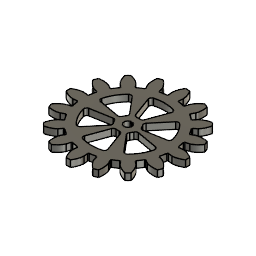
Gear 1 (Autodesk Fusion 360 design; units mm, degrees)
description: Spur Gear; Module: 12.700000; Num Teeth: 16; Pressure Angle: 20.000000; Backlash: 0.00 mm
Autodesk Fusion 360 part; units mm, degrees
sketch "Sketch1" plane through (0, 0, 0) normal (0, 0, 1) x (1, 0, 0) in component "Spur Gear (16 teeth)"
  circle A0 centre (0, 0) radius 86.3092
  circle A1 centre (0, 0) radius 6.35
extrude "Extrude1" add sketch "Sketch1" along normal blind 12.7 in component "Spur Gear (16 teeth)"
sketch "Sketch2" plane through (0, 0, 0) normal (0, 0, 1) x (1, 0, 0) in component "Spur Gear (16 teeth)"
  spline S0 degree 5 poles (94.863, -10.773) (94.919, -10.7793) (95.0311, -10.7904) (95.1995, -10.8021) (95.4243, -10.8085) (95.706, -10.8038) (95.9881, -10.7901) (96.2705, -10.7709) (96.5529, -10.7488) (96.8354, -10.7247) (97.1179, -10.6983) (97.4005, -10.669) (97.683, -10.6358) (97.9655, -10.5982) (98.2481, -10.5561) (98.5306, -10.51) (98.813, -10.4605) (99.0953, -10.4081) (99.3775, -10.3532) (99.6596, -10.2959) (99.9416, -10.2361) (100.2234, -10.1738) (100.505, -10.1088) (100.7865, -10.041) (101.0678, -9.9705) (101.3489, -9.8975) (101.6299, -9.8219) (101.9106, -9.7441) (102.1911, -9.664) (102.4714, -9.5816) (102.7515, -9.4971) (103.0313, -9.4104) (103.3109, -9.3215) (103.5902, -9.2304) (103.8693, -9.1372) (104.1481, -9.0418) (104.4266, -8.9443) (104.7048, -8.8449) (104.9828, -8.7434) (105.2604, -8.6399) (105.5378, -8.5345) (105.8149, -8.4272) (106.0916, -8.3179) (106.368, -8.2067) (106.6441, -8.0937) (106.9199, -7.9787) (107.1953, -7.8619) (107.4704, -7.7433) (107.7452, -7.6229) (108.0196, -7.5007) (108.2936, -7.3767) (108.5673, -7.2509) (108.8406, -7.1234) (109.1135, -6.9942) (109.3861, -6.8632) (109.6583, -6.7306) (109.93, -6.5962) (110.2014, -6.4602) (110.4724, -6.3225) (110.743, -6.1831) (111.0132, -6.0422) (111.283, -5.8995) (111.5523, -5.7553) (111.8213, -5.6095) (112.0898, -5.4621) (112.3578, -5.3131) (112.6255, -5.1625) (112.8927, -5.0104) (113.1594, -4.8567) (113.4257, -4.7015) (113.6916, -4.5447) (113.9039, -4.4181) (114.063, -4.3224) (114.1689, -4.2584) (114.2218, -4.2262) knots 0 0 0 0 0 0 0.01428571 0.02857143 0.04285714 0.05714286 0.07142857 0.08571429 0.1 0.11428571 0.12857143 0.14285714 0.15714286 0.17142857 0.18571429 0.2 0.21428571 0.22857143 0.24285714 0.25714286 0.27142857 0.28571429 0.3 0.31428571 0.32857143 0.34285714 0.35714286 0.37142857 0.38571429 0.4 0.41428571 0.42857143 0.44285714 0.45714286 0.47142857 0.48571429 0.5 0.51428571 0.52857143 0.54285714 0.55714286 0.57142857 0.58571429 0.6 0.61428571 0.62857143 0.64285714 0.65714286 0.67142857 0.68571429 0.7 0.71428571 0.72857143 0.74285714 0.75714286 0.77142857 0.78571429 0.8 0.81428571 0.82857143 0.84285714 0.85714286 0.87142857 0.88571429 0.9 0.91428571 0.92857143 0.94285714 0.95714286 0.97142857 0.98571429 1 1 1 1 1 1
  spline S1 degree 5 poles (94.863, 10.773) (94.919, 10.7793) (95.0311, 10.7904) (95.1995, 10.8021) (95.4243, 10.8085) (95.706, 10.8038) (95.9881, 10.7901) (96.2705, 10.7709) (96.5529, 10.7488) (96.8354, 10.7247) (97.1179, 10.6983) (97.4005, 10.669) (97.683, 10.6358) (97.9655, 10.5982) (98.2481, 10.5561) (98.5306, 10.51) (98.813, 10.4605) (99.0953, 10.4081) (99.3775, 10.3532) (99.6596, 10.2959) (99.9416, 10.2361) (100.2234, 10.1738) (100.505, 10.1088) (100.7865, 10.041) (101.0678, 9.9705) (101.3489, 9.8975) (101.6299, 9.8219) (101.9106, 9.7441) (102.1911, 9.664) (102.4714, 9.5816) (102.7515, 9.4971) (103.0313, 9.4104) (103.3109, 9.3215) (103.5902, 9.2304) (103.8693, 9.1372) (104.1481, 9.0418) (104.4266, 8.9443) (104.7048, 8.8449) (104.9828, 8.7434) (105.2604, 8.6399) (105.5378, 8.5345) (105.8149, 8.4272) (106.0916, 8.3179) (106.368, 8.2067) (106.6441, 8.0937) (106.9199, 7.9787) (107.1953, 7.8619) (107.4704, 7.7433) (107.7452, 7.6229) (108.0196, 7.5007) (108.2936, 7.3767) (108.5673, 7.2509) (108.8406, 7.1234) (109.1135, 6.9942) (109.3861, 6.8632) (109.6583, 6.7306) (109.93, 6.5962) (110.2014, 6.4602) (110.4724, 6.3225) (110.743, 6.1831) (111.0132, 6.0422) (111.283, 5.8995) (111.5523, 5.7553) (111.8213, 5.6095) (112.0898, 5.4621) (112.3578, 5.3131) (112.6255, 5.1625) (112.8927, 5.0104) (113.1594, 4.8567) (113.4257, 4.7015) (113.6916, 4.5447) (113.9039, 4.4181) (114.063, 4.3224) (114.1689, 4.2584) (114.2218, 4.2262) knots 0 0 0 0 0 0 0.01428571 0.02857143 0.04285714 0.05714286 0.07142857 0.08571429 0.1 0.11428571 0.12857143 0.14285714 0.15714286 0.17142857 0.18571429 0.2 0.21428571 0.22857143 0.24285714 0.25714286 0.27142857 0.28571429 0.3 0.31428571 0.32857143 0.34285714 0.35714286 0.37142857 0.38571429 0.4 0.41428571 0.42857143 0.44285714 0.45714286 0.47142857 0.48571429 0.5 0.51428571 0.52857143 0.54285714 0.55714286 0.57142857 0.58571429 0.6 0.61428571 0.62857143 0.64285714 0.65714286 0.67142857 0.68571429 0.7 0.71428571 0.72857143 0.74285714 0.75714286 0.77142857 0.78571429 0.8 0.81428571 0.82857143 0.84285714 0.85714286 0.87142857 0.88571429 0.9 0.91428571 0.92857143 0.94285714 0.95714286 0.97142857 0.98571429 1 1 1 1 1 1
  arc A0 (114.2218, -4.2262) -> (114.2218, 4.2262) centre (0, 0) ccw
  line L0 (85.748, -9.739) -> (94.863, -10.773)
  line L1 (85.748, 9.739) -> (94.863, 10.773)
  line L2 (85.748, -9.739) -> (85.748, 9.739)
  point P0 (96.2162, -10.774)
  point P1 (97.5833, -10.647)
  point P2 (98.9587, -10.4331)
  point P3 (100.3403, -10.1465)
  point P4 (101.7263, -9.7949)
  point P5 (103.1155, -9.3833)
  point P6 (104.5068, -8.9153)
  point P7 (105.8991, -8.3936)
  point P8 (107.2914, -7.8202)
  point P9 (108.6828, -7.1968)
  point P10 (110.0724, -6.5246)
  point P11 (111.4593, -5.8049)
  point P12 (112.8428, -5.0385)
  point P13 (96.2162, 10.774)
  point P14 (97.5833, 10.647)
  point P15 (98.9587, 10.4331)
  point P16 (100.3403, 10.1465)
  point P17 (101.7263, 9.7949)
  point P18 (103.1155, 9.3833)
  point P19 (104.5068, 8.9153)
  point P20 (105.8991, 8.3936)
  point P21 (107.2914, 7.8202)
  point P22 (108.6828, 7.1968)
  point P23 (110.0724, 6.5246)
  point P24 (111.4593, 5.8049)
  point P25 (112.8428, 5.0385)
extrude "Extrude2" add sketch "Sketch2" along normal blind 12.7 in component "Spur Gear (16 teeth)"
fillet "Fillet1" radius 1.5875 2 edges at (85.7578, -9.7401, 6.35) (85.7578, 9.7401, 6.35) in component "Spur Gear (16 teeth)"
pattern_circular "C-Pattern1" count 16 over 360 about axis through (0, 0, 0) along (0, 0, 1) of "Extrude2", "Fillet1" in component "Spur Gear (16 teeth)"
sketch "Sketch3" plane through (0, 0, 0) normal (0, 0, 1) x (1, 0, 0) in component "Spur Gear (16 teeth)"
  circle A0 centre (0, 0) radius 101.6 construction
sketch "Sketch1 (2)" plane through (0, 0, 0) normal (0, 0, 1) x (1, 0, 0)
  circle A0 centre (0, 0) radius 7.55
  line L0 (0, 13) -> (0, -11)
  line L1 (1.4, 7.4191) -> (1.4, 5.65)
  line L2 (1.4, 5.65) -> (-1.4, 5.65)
  line L3 (-1.4, 5.65) -> (-1.4, 7.4191)
  circle A1 centre (0, 0) radius 70
  circle A2 centre (0, 0) radius 20
  line L4 (0, 0) -> (-6.8404, 18.7939)
  line L5 (0, 0) -> (6.8404, 18.7939)
  line L6 (-6.8404, 18.7939) -> (-23.9414, 65.7785)
  line L7 (6.8404, 18.7939) -> (23.9414, 65.7785)
  line L8 (-19.6962, 3.473) -> (-68.9365, 12.1554)
  line L9 (-12.8558, 15.3209) -> (-44.9951, 53.6231)
  line L10 (-12.8558, -15.3209) -> (-44.9951, -53.6231)
  line L11 (-19.6962, -3.473) -> (-68.9365, -12.1554)
  line L12 (6.8404, -18.7939) -> (23.9414, -65.7785)
  line L13 (-6.8404, -18.7939) -> (-23.9414, -65.7785)
  line L14 (19.6962, -3.473) -> (68.9365, -12.1554)
  line L15 (12.8558, -15.3209) -> (44.9951, -53.6231)
  line L16 (12.8558, 15.3209) -> (44.9951, 53.6231)
  line L17 (19.6962, 3.473) -> (68.9365, 12.1554)
  point P0 (0, 7.55)
  dimension "d17" = 15.1
  dimension "d18" = 2.8
  dimension "d19" = 1.9
  dimension "d24" = -50
  dimension "d25" = 40
  dimension "d26" = 40
  dimension "d28" = 20
  dimension "d30" = 360
  constraint coincident A0.centre A1.centre
  constraint vertical L0
  constraint coincident A0 L1.start
  constraint parallel L0 L1
  constraint perpendicular L0 L2
  constraint perpendicular L2 L3
  constraint coincident A0 L3.end
  constraint coincident A0 P0
  constraint coincident L0 P0
  constraint coincident A0.centre L0
  constraint concentric A0 A1
  constraint coincident A1 L6.end
  constraint coincident A1 L7.end
  constraint coincident A2 L4.end
  constraint coincident A2 L5.end
  measures "d17" diameter of A0
  measures "d18" distance of L1 L3
  measures "d19" distance of L2 P0
  measures "d25" diameter of A2
  measures "d26" angle of L4 L5
  measures "d28" angle of L0 L5
extrude "Extrude3" cut sketch "Sketch1 (2)" along normal up to surface (12.7 mm away) contours A0 L0 L5 | A0 L0 L1 L2 L5 | A0 L0 L4 | A0 L0 L2 L3 L4 in component "Spur Gear (16 teeth)"
extrude "Extrude4" add sketch "Sketch1 (2)" along normal up to surface (12.7 mm away) contours A0 L0 L1 L2 | A0 L0 L2 L3 in component "Spur Gear (16 teeth)"
extrude "Extrude5" cut sketch "Sketch1 (2)" along normal up to surface (12.7 mm away) contours A1 A2 L6 L7 | A1 A2 L16 L17 | A1 A2 L8 L9 | A1 A2 L14 L15 | A1 A2 L10 L11 | A1 A2 L12 L13 in component "Spur Gear (16 teeth)"
fillet "Fillet2" radius 5 12 edges at (23.9414, 65.7785, 6.35) (-23.9414, 65.7785, 6.35) (44.9951, 53.6231, 6.35) (68.9365, 12.1554, 6.35) (68.9365, -12.1554, 6.35) (44.9951, -53.6231, 6.35) (23.9414, -65.7785, 6.35) (-44.9951, -53.6231, 6.35) (-23.9414, -65.7785, 6.35) (-68.9365, -12.1554, 6.35) (-68.9365, 12.1554, 6.35) (-44.9951, 53.6231, 6.35) in component "Spur Gear (16 teeth)"
fillet "Fillet2" radius 5 12 edges at (-19.6962, 3.473, 6.35) (-12.8558, 15.3209, 6.35) (-19.6962, -3.473, 6.35) (-12.8558, -15.3209, 6.35) (-6.8404, -18.7939, 6.35) (6.8404, -18.7939, 6.35) (12.8558, -15.3209, 6.35) (19.6962, -3.473, 6.35) (19.6962, 3.473, 6.35) (12.8558, 15.3209, 6.35) (6.8404, 18.7939, 6.35) (-6.8404, 18.7939, 6.35) in component "Spur Gear (16 teeth)"
component "Spur Gear (16 teeth)" placed x (1, 0, 0) y (0, 1, 0) z (0, 0, 1) at (0, 0, 0)
